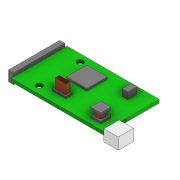
# Autodesk Inventor part: Nano-modem
Saved by Autodesk Inventor 2022.3 (Build 263350000, 350)
## iProperties
Created: 2023-07-18
Part Number: Nano-modem
Material: Genérico
Document SubType Name: Modeling
Designer: Usuario
Density: 1 g/cm^3
Appearance: Valor por defecto
Author: Usuario
Autodesk Inventor part; units mm, degrees
ref_plane "YZ Plane" through (0, 0, 0) normal (1, 0, 0) x (0, 1, 0)
ref_plane "XZ Plane" through (0, 0, 0) normal (0, 1, 0) x (-1, 0, 0)
ref_plane "XY Plane" through (0, 0, 0) normal (0, 0, 1) x (1, 0, 0)
sketch "Boceto1" plane through (0, 0, 0) normal (0, 1, 0) x (-1, 0, 0)
  line L0 (-22.5, 13.55) -> (22.5, 13.55)
  line L1 (22.5, 13.55) -> (22.5, -13.55)
  line L2 (22.5, -13.55) -> (-22.5, -13.55)
  line L3 (-22.5, -13.55) -> (-22.5, 13.55)
  line L4 (-22.5, 13.55) -> (22.5, -13.55) construction
  line L5 (22.5, 13.55) -> (-22.5, -13.55) construction
  line L6 (22.5, 0) -> (12.5, 0)
  line L7 (12.5, 0) -> (12.5, 10)
  line L8 (12.5, 10) -> (12.5, -10)
  circle A0 centre (12.5, 10) radius 1.5
  circle A1 centre (12.5, -10) radius 1.5
  point P0 (0, 0)
  dimension "d0" = 45
  dimension "d1" = 27.1
  dimension "d2" = 10
  dimension "d3" = 10
  dimension "d4" = 20
  dimension "d5" = 3
  dimension "d6" = 3
  constraints: 18 end point, 3 midpoint, 2 centre point, 2 coincident, 2 horizontal, 2 parallel, 1 perpendicular, 1 point on line, 1 vertical
  measures "d0" distance of L1.end L2.end
  measures "d1" distance of L0.end L1.end
  measures "d2" distance of L6.start L6.end
  measures "d3" distance of L6.end L7.end
  measures "d4" distance of L7.end L8.end
  measures "d5" diameter of A0
  measures "d6" diameter of A1
extrude "Extrusión1" add sketch "Boceto1" along normal blind 1.6
sketch "Boceto2" plane through (-22.5, 0, -13.55) normal (-1, 0, 0) x (0, 0, 1)
  line L0 (13.55, 0) -> (13.55, 1.6)
  line L1 (27.1, 1.6) -> (0, 1.6) projected
  line L2 (26.05, -1.7) -> (1.05, -1.7)
  line L3 (1.05, -1.7) -> (1.05, 3.3)
  line L4 (1.05, 3.3) -> (26.05, 3.3)
  line L5 (26.05, 3.3) -> (26.05, -1.7)
  line L6 (26.05, -1.7) -> (1.05, 3.3) construction
  line L7 (1.05, -1.7) -> (26.05, 3.3) construction
  point P0 (13.55, 0.8)
  dimension "d9" = 25
  dimension "d10" = 5
  constraints: 14 end point, 4 midpoint, 2 parallel, 1 horizontal, 1 perpendicular
  measures "d9" distance of L3.end L4.end
  measures "d10" distance of L2.end L3.end
extrude "Extrusión2" add sketch "Boceto2" along normal blind 2.5
sketch "Boceto3" plane through (22.5, 0, 13.55) normal (1, 0, 0) x (0, 0, -1)
  line L0 (0, 2.7012) -> (7.5, 2.7012)
  line L1 (7.5, 2.7012) -> (7.5, -2.8988)
  line L2 (7.5, -2.8988) -> (0, -2.8988)
  line L3 (0, -2.8988) -> (0, 2.7012)
  point P0 (13.55, 0)
  dimension "d13" = 7.5
  dimension "d14" = 5.6
  constraints: 8 end point, 2 parallel, 1 horizontal, 1 perpendicular
  measures "d13" distance of L1.end L2.end
  measures "d14" distance of L0.end L1.end
extrude "Extrusión3" add sketch "Boceto3" along normal blind 7
sketch "Boceto4" plane through (0, 1.6, 0) normal (0, 1, 0) x (1, 0, 0)
  line L0 (-8.6118, -0.6728) -> (1.3882, -0.6728)
  line L1 (1.3882, -0.6728) -> (1.3882, 9.3272)
  line L2 (1.3882, 9.3272) -> (-8.6118, 9.3272)
  line L3 (-8.6118, 9.3272) -> (-8.6118, -0.6728)
  line L4 (-7.0868, -9.0155) -> (-0.5382, -9.0155)
  line L5 (-0.5382, -9.0155) -> (-0.5382, -5.8757)
  line L6 (-0.5382, -5.8757) -> (-7.0868, -5.8757)
  line L7 (-7.0868, -5.8757) -> (-7.0868, -9.0155)
  line L8 (12.2897, 5.6963) -> (14.9809, 5.6963)
  line L9 (14.9809, 5.6963) -> (14.9809, 10.0919)
  line L10 (14.9809, 10.0919) -> (12.2897, 10.0919)
  line L11 (12.2897, 10.0919) -> (12.2897, 5.6963)
  line L12 (13.6353, -11.1684) -> (18.6353, -11.1684)
  line L13 (18.6353, -11.1684) -> (18.6353, -6.1684)
  line L14 (18.6353, -6.1684) -> (13.6353, -6.1684)
  line L15 (13.6353, -6.1684) -> (13.6353, -11.1684)
  point P0 (0, 0)
  dimension "d17" = 10
  dimension "d18" = 10
  dimension "d19" = 5
  dimension "d20" = 5
  constraints: 32 end point, 8 parallel, 4 horizontal, 4 perpendicular
  measures "d17" distance of L2.end L1.end
  measures "d18" distance of L1.end L0.end
  measures "d19" distance of L14.end L13.end
  measures "d20" distance of L13.end L12.end
extrude "Extrusión4" add sketch "Boceto4" along normal blind 1
sketch "Boceto5" plane through (0, 2.6, 0) normal (0, 1, 0) x (1, 0, 0)
  line L0 (-6.3329, -8.4587) -> (-1.0802, -8.4587)
  line L1 (-1.0802, -8.4587) -> (-1.0802, -6.3765)
  line L2 (-1.0802, -6.3765) -> (-6.3329, -6.3765)
  line L3 (-6.3329, -6.3765) -> (-6.3329, -8.4587)
  point P0 (0, 0)
  constraints: 8 end point, 2 parallel, 1 horizontal, 1 perpendicular
extrude "Extrusión5" add sketch "Boceto5" along normal blind 4.7
sketch "Boceto6" plane through (0, 2.6, 0) normal (0, 1, 0) x (1, 0, 0)
  circle A0 centre (16.0574, -8.6684) radius 1.8966
  point P0 (0, 0)
  constraints: 1 centre point
extrude "Extrusión6" add sketch "Boceto6" along normal blind 2.7
sketch "Boceto7" plane through (16.0574, 5.3, 8.6684) normal (0, 1, 0) x (1, 0, 0)
  circle A0 centre (0, 0) radius 1.8966 projected
  line L0 (2.5779, -2.5) -> (2.5779, 2.5) projected
  line L1 (2.5779, 2.5) -> (-2.4221, 2.5) projected
  line L2 (-2.4221, 2.5) -> (-2.4221, -2.5) projected
  line L3 (-2.4221, -2.5) -> (2.5779, -2.5) projected
  circle A1 centre (0, 0) radius 1.8966 projected
  point P0 (-16.0574, 8.6684)
extrude "Extrusión7" add sketch "Boceto7" along normal blind 1 contours A0 | L3 L2 L1 L0
sketch "Boceto8" plane through (0, 2.6, 0) normal (0, 1, 0) x (1, 0, 0)
  line L0 (14.9809, 5.6963) -> (14.9809, 10.0919) projected
  line L1 (14.9809, 10.0919) -> (12.2897, 10.0919) projected
  line L2 (12.2897, 10.0919) -> (12.2897, 5.6963) projected
  line L3 (12.2897, 5.6963) -> (14.9809, 5.6963) projected
  point P0 (0, 0)
extrude "Extrusión8" add sketch "Boceto8" along normal blind 2.3
sketch "Boceto9" plane through (-22.5, 0, 13.55) normal (0, 0, 1) x (1, 0, 0)
  line L0 (52, -2.8988) -> (52, 2.7012) projected
  line L1 (45, -2.8988) -> (52, -2.8988) projected
  line L2 (52, 2.7012) -> (45, 2.7012)
  line L3 (45, 2.7012) -> (45, -2.8988)
  line L4 (45, -2.8988) -> (52, -2.8988)
  line L5 (52, -2.8988) -> (52, 2.7012)
  point P0 (22.5, 0)
  constraints: 8 end point, 2 parallel, 1 horizontal, 1 perpendicular
extrude "Extrusión9" cut sketch "Boceto9" against normal blind 0.1
